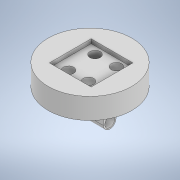
# Autodesk Inventor part: shaft_mount_wrist
Saved by Autodesk Inventor 2022 (Build 260153000, 153)
## iProperties
Created: 2022-01-29
Part Number: shaft_mount_wrist
Material: Generic
Document SubType Name: Modeling
Designer: pauly
Density: 1 g/cm^3
Appearance: Default
Author: pauly
Autodesk Inventor part; units mm, degrees
ref_plane "YZ Plane" through (0, 0, 0) normal (1, 0, 0) x (0, 1, 0)
ref_plane "XZ Plane" through (0, 0, 0) normal (0, 1, 0) x (-1, 0, 0)
ref_plane "XY Plane" through (0, 0, 0) normal (0, 0, 1) x (1, 0, 0)
sketch "Sketch1" plane through (0, 0, 0) normal (1, 0, 0) x (0, 1, 0)
  circle A0 centre (0, 0) radius 2.9972
  arc A1 (0, 3.81) -> (0, -3.81) centre (0, 0) ccw
  line L0 (0, 3.81) -> (12.7, 3.81)
  line L1 (0, -3.81) -> (12.7, -3.81)
  line L2 (12.7, -3.81) -> (12.7, 3.81)
  dimension "d0" = 5.9944
  dimension "d4" = 7.62
  dimension "d5" = 12.7
  dimension "d6" = 12.7
  constraints: 6 end point, 2 centre point, 2 horizontal, 2 point on circle, 1 coincident, 1 perpendicular
  measures "d0" diameter of A0
  measures "d4" diameter of A1
  measures "d5" distance of L0.start L0.end
  measures "d6" distance of L1.start L1.end
extrude "Extrusion1" add sketch "Sketch1" along normal blind 24.003
sketch "Sketch2" plane through (0, 12.7, 3.81) normal (0, 1, 0) x (1, 0, 0)
  line L0 (0, 7.62) -> (24.003, 7.62) projected
  circle A0 centre (12.0015, 3.81) radius 25.4
  point P0 (0, 3.81)
  dimension "d9" = 50.8
  constraints: 1 centre point
  measures "d9" diameter of A0
extrude "Extrusion2" add sketch "Sketch2" along normal blind 12.7
sketch "Sketch3" plane through (12.0015, 25.4, 0) normal (0, 1, 0) x (1, 0, 0)
  line L0 (-12.0015, 2.9972) -> (-12.0015, -2.9972) projected
  line L1 (-12.0015, -12.7) -> (-12.0015, 12.7)
  line L2 (-12.0015, -12.7) -> (13.3985, -12.7)
  line L3 (13.3985, -12.7) -> (13.3985, 12.7)
  line L4 (13.3985, 12.7) -> (-12.0015, 12.7)
  line L5 (-12.0015, 12.7) -> (-12.0015, -12.7)
  circle A0 centre (-5.6515, -8.128) radius 1.905
  line L6 (13.3985, -12.7) -> (13.3985, -8.128)
  line L7 (13.3985, -12.7) -> (13.3985, -8.128)
  line L8 (13.3985, -12.7) -> (13.3985, -8.128)
  circle A1 centre (7.0485, -8.128) radius 1.905
  circle A2 centre (-5.6515, 8.128) radius 1.905
  circle A3 centre (7.0485, 8.128) radius 1.905
  circle A4 centre (-5.6515, -8.128) radius 1.905
  circle A5 centre (7.0485, -8.128) radius 1.905
  point P0 (-12.0015, 0)
  dimension "d13" = 25.4
  dimension "d14" = 25.4
  dimension "d17" = 3.81
  dimension "d20" = 3.81
  dimension "d23" = 3.81
  dimension "d24" = 3.81
  dimension "d25" = 3.81
  dimension "d26" = 3.81
  constraints: 16 end point, 6 centre point, 2 parallel, 1 collinear, 1 horizontal, 1 perpendicular, 1 point on line, 1 vertical
  measures "d13" distance of L1.start L1.end
  measures "d14" distance of L4.end L3.end
  measures "d17" diameter of A0
  measures "d20" diameter of A1
  measures "d23" diameter of A2
  measures "d24" diameter of A3
  measures "d25" diameter of A4
  measures "d26" diameter of A5
extrude "Extrusion3" cut sketch "Sketch3" against normal blind 2.54
sketch "Sketch4" plane through (6.35, 25.4, 8.128) normal (0, 1, 0) x (1, 0, 0)
  point P0 (-6.35, 8.128)
  point P1 (0.8022, -0.041)
hole "Hole1" at (7.1522, 25.4, 8.169) direction (0, -1, 0) diameter 6.35 end through all
sketch "Sketch5" plane through (6.35, 25.4, -8.128) normal (0, 1, 0) x (1, 0, 0)
  point P0 (-6.35, -8.128)
  point P1 (0.6252, -0.0267)
  point P2 (13.4879, 0.0841)
  point P3 (12.7137, -16.0745)
hole "Hole2" at (6.9752, 25.4, -8.1013) at (19.8379, 25.4, -8.2121) at (19.0637, 25.4, 7.9465) direction (0, -1, 0) diameter 6.35 end through all
body "Solid1"
